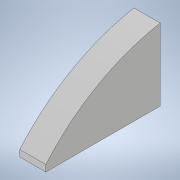
# Autodesk Inventor part: FP Cockpit
Saved by Autodesk Inventor 2020 (Build 240168000, 168)
## iProperties
Created: 2021-04-23
Part Number: FP Cockpit
Material: Generic
Document SubType Name: Modeling
Designer: austi
Density: 1 g/cm^3
Appearance: Default
Author: austi
Autodesk Inventor part; units mm, degrees
ref_plane "YZ Plane" through (0, 0, 0) normal (1, 0, 0) x (0, 1, 0)
ref_plane "XZ Plane" through (0, 0, 0) normal (0, 1, 0) x (-1, 0, 0)
ref_plane "XY Plane" through (0, 0, 0) normal (0, 0, 1) x (1, 0, 0)
sketch "Sketch1" plane through (0, 0, 0) normal (0, 1, 0) x (-1, 0, 0)
  line L0 (0, 0) -> (0, -35)
  line L1 (0, 0) -> (22, 0)
  line L2 (0, -35) -> (2, -35)
  line L3 (0, -17.5) -> (16, -17.5)
  arc A0 (2, -35) -> (22, 0) centre (-36.7812, 10.375) ccw
  dimension "d0" = 35
  dimension "d1" = 22
  dimension "d2" = 2
  dimension "d3" = 16
  constraints: 8 end point, 3 horizontal, 3 point on circle, 1 centre point, 1 midpoint, 1 vertical
  measures "d0" distance of L0.start L0.end
  measures "d1" distance of L0.start L1.end
  measures "d2" distance of L0.end L2.end
  measures "d3" distance of L3.start L3.end
extrude "Extrusion1" add sketch "Sketch1" along normal blind 8
body "Solid1"
